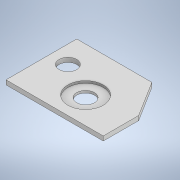
# Autodesk Inventor part: GuidePlate
Saved by Autodesk Inventor 2022.2 (Build 262287030, 287C)
## iProperties
Created: 2023-02-22
Part Number: GuidePlate
Material: Generic
Document SubType Name: Modeling
Designer: jak27277
Density: 1 g/cm^3
Appearance: Default
Author: jak27277
Autodesk Inventor part; units mm, degrees
ref_plane "YZ Plane" through (0, 0, 0) normal (1, 0, 0) x (0, 1, 0)
ref_plane "XZ Plane" through (0, 0, 0) normal (0, 1, 0) x (-1, 0, 0)
ref_plane "XY Plane" through (0, 0, 0) normal (0, 0, 1) x (1, 0, 0)
sketch "Sketch1" plane through (0, 0, 0) normal (0, 1, 0) x (-1, 0, 0)
  line L0 (0, 0) -> (-139.7, 0)
  line L1 (-107.95, -101.6) -> (0, -101.6)
  line L2 (0, -101.6) -> (0, 0)
  line L3 (-107.95, -101.6) -> (-139.7, -50.8)
  line L4 (-139.7, -50.8) -> (-139.7, 0)
  circle A0 centre (-25.4, -63.5) radius 12.7
  circle A1 centre (-76.2, -38.1) radius 12.7
  dimension "d0" = 50.8
  dimension "d1" = 101.6
  dimension "d2" = 107.95
  dimension "d3" = 139.7
  dimension "d5" = 25.4
  dimension "d6" = 63.5
  dimension "d7" = 38.1
  dimension "d8" = 76.2
  dimension "d9" = 25.4
  constraints: 10 end point, 2 centre point, 2 vertical, 1 equal radius, 1 horizontal, 1 parallel
  measures "d0" distance of L3.end L0.end
  measures "d1" distance of L1.end L0.start
  measures "d2" distance of L1.start L1.end
  measures "d3" distance of L0.start L0.end
  measures "d5" distance from line of A0.centre L2
  measures "d6" distance from line of L0 A0.centre
  measures "d7" distance from line of L0 A1.centre
  measures "d8" distance from line of L2 A1.centre
  measures "d9" diameter of A0
extrude "Extrusion1" add sketch "Sketch1" along normal blind 6.35
sketch "Sketch2" plane through (0, 6.35, 0) normal (0, 1, 0) x (1, 0, 0)
  circle A0 centre (76.2, 38.1) radius 12.7 projected
  point P0 (0, 0)
  constraints: 1 coincident
hole "Hole1" at (76.2, 6.35, -38.1) direction (0, -1, 0) diameter 25.4 end through all counterbore diameter 50.8 counterbore depth 3.175
body "Solid1"
